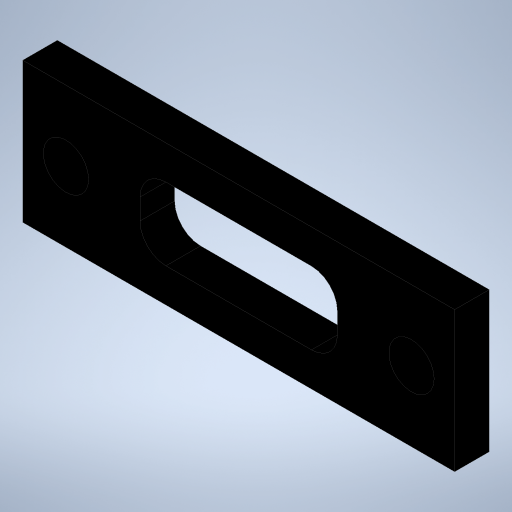
# Autodesk Inventor part: USB-C_face_plate
Saved by Autodesk Inventor 2024 (Build 280153000, 153)
## iProperties
Created: 2026-04-14
Part Number: USB-C_face_plate
Material: Generic
Document SubType Name: Modeling
Designer: Login
Density: 1 g/cm^3
Appearance: Default
Author: Login
Autodesk Inventor part; units mm, degrees
ref_plane "YZ Plane" through (0, 0, 0) normal (1, 0, 0) x (0, 1, 0)
ref_plane "XZ Plane" through (0, 0, 0) normal (0, 1, 0) x (-1, 0, 0)
ref_plane "XY Plane" through (0, 0, 0) normal (0, 0, 1) x (1, 0, 0)
sketch "Sketch1" plane through (0, 0, 0) normal (0, 0, 1) x (1, 0, 0)
  line L0 (-10, 3.25) -> (10, 3.25)
  line L1 (10, 3.25) -> (10, -3.25)
  line L2 (10, -3.25) -> (-10, -3.25)
  line L3 (-10, -3.25) -> (-10, 3.25)
  line L4 (-10, 3.25) -> (10, -3.25) construction
  line L5 (10, 3.25) -> (-10, -3.25) construction
  point P0 (0, 0)
  dimension "d0" = 20
  dimension "d1" = 6.5
  constraints: 12 end point, 2 midpoint, 2 parallel, 1 horizontal, 1 perpendicular
  measures "d0" distance of L1.end L2.end
  measures "d1" distance of L0.end L1.end
extrude "Extrusion1" add sketch "Sketch1" along normal blind 1.6
sketch "Sketch2" plane through (0, 0, 1.6) normal (0, 0, 1) x (1, 0, 0)
  line L0 (10, -3.25) -> (10, 3.25) projected
  line L1 (-10, 3.25) -> (-10, -3.25) projected
  line L2 (10, 3.25) -> (-10, 3.25) projected
  point P0 (0, 0)
  point P1 (-8, 0)
  point P2 (8, 0)
  dimension "d4" = 2
  dimension "d5" = 2
  dimension "d6" = 3.25
  dimension "d7" = 3.25
  measures "d4" distance from line of L0 point (8, 0)
  measures "d5" distance from line of L1 point (-8, 0)
  measures "d6" distance from line of L2 point (-8, 0)
  measures "d7" distance from line of L2 point (8, 0)
hole "Hole1" at (-8, 0, 1.6) at (8, 0, 1.6) direction (0, 0, -1) diameter 2.1 end through all
sketch "Sketch3" plane through (0, 0, 1.6) normal (0, 0, 1) x (1, 0, 0)
  line L0 (-3.37, 1.68) -> (3.37, 1.68)
  line L1 (4.57, 0.48) -> (4.57, -0.48)
  line L2 (3.37, -1.68) -> (-3.37, -1.68)
  line L3 (-4.57, -0.48) -> (-4.57, 0.48)
  line L4 (-4.57, 1.68) -> (4.57, -1.68) construction
  line L5 (4.57, 1.68) -> (-4.57, -1.68) construction
  arc A0 (-3.37, 1.68) -> (-4.57, 0.48) centre (-3.37, 0.48) ccw
  arc A1 (4.57, 0.48) -> (3.37, 1.68) centre (3.37, 0.48) ccw
  arc A2 (3.37, -1.68) -> (4.57, -0.48) centre (3.37, -0.48) ccw
  arc A3 (-4.57, -0.48) -> (-3.37, -1.68) centre (-3.37, -0.48) ccw
  point P0 (0, 0)
  point P1 (-4.57, 0)
  point P2 (4.57, 0)
  dimension "d15" = 9.14
  dimension "d16" = 3.36
  dimension "d17" = 1.2
  constraints: 12 end point, 8 point on circle, 8 point on line, 8 tangent, 4 centre point, 3 equal radius, 2 midpoint, 2 parallel, 1 horizontal, 1 perpendicular
  measures "d15" distance of L4.end L5.end
  measures "d16" distance of L5.start L4.end
  measures "d17" radius of A0
extrude "Extrusion2" cut sketch "Sketch3" against normal blind 1.6
body "Solid1"
